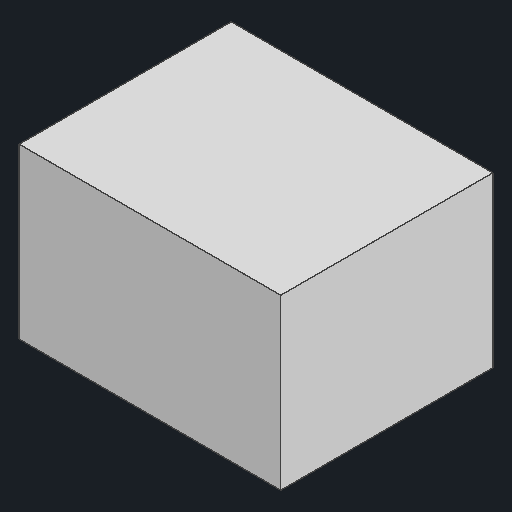
# Autodesk Inventor part: XznyCompactSeriesX
Saved by Autodesk Inventor 2025.2 (Build 292293000, 293)
## iProperties
Created: 2025-11-05
Part Number: XznyCompactSeriesX
Material: Generic
Document SubType Name: Modeling
Designer: valer
Density: 1 g/cm^3
Appearance: Default
Author: valer
Autodesk Inventor part; units mm, degrees
ref_plane "YZ Plane" through (0, 0, 0) normal (1, 0, 0) x (0, 1, 0)
ref_plane "XZ Plane" through (0, 0, 0) normal (0, 1, 0) x (-1, 0, 0)
ref_plane "XY Plane" through (0, 0, 0) normal (0, 0, 1) x (1, 0, 0)
sketch "Sketch1" plane through (0, 0, 0) normal (0, 0, 1) x (1, 0, 0)
  line L0 (130.048, -83.947) -> (-130.048, -83.947)
  line L1 (-130.048, -83.947) -> (-130.048, 83.947)
  line L2 (-130.048, 83.947) -> (130.048, 83.947)
  line L3 (130.048, 83.947) -> (130.048, -83.947)
  line L4 (130.048, -83.947) -> (-130.048, 83.947) construction
  line L5 (-130.048, -83.947) -> (130.048, 83.947) construction
  point P0 (0, 0)
  dimension "d0" = 260.096
  dimension "d1" = 167.894
  constraints: 12 end point, 2 midpoint, 2 parallel, 1 horizontal, 1 perpendicular
  measures "d0" distance of L1.end L2.end
  measures "d1" distance of L2.end L0.start
extrude "Extrusion1" add sketch "Sketch1" along normal blind 210.82
body "Solid1"
